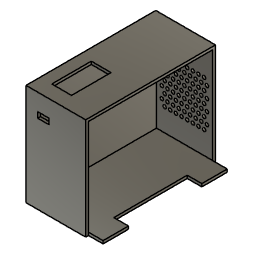
Pc v2.1 v3 (Autodesk Fusion 360 design; units mm, degrees)
Autodesk Fusion 360 part; units mm, degrees
sketch "Boceto1" plane through (0, 0, 0) normal (1, 0, 0) x (0, 1, 0)
  line L0 (0, 0) -> (230, 0)
  line L1 (230, 0) -> (230, 180)
  line L2 (230, 180) -> (0, 180)
  line L3 (0, 180) -> (0, 0)
  line L4 (5, 5) -> (225, 5)
  line L5 (225, 5) -> (225, 175)
  line L6 (225, 175) -> (5, 175)
  line L7 (5, 175) -> (5, 5)
  constraint horizontal L0
  constraint vertical L1
  constraint horizontal L2
  constraint vertical L3
  constraint coincident L0.start L3.end
  constraint horizontal L4
  constraint vertical L5
  constraint horizontal L6
  constraint vertical L7
extrude "Extruir1" add sketch "Boceto1" along normal blind 100
sketch "Boceto2" plane through (0, 230, 0) normal (0, 1, 0) x (-1, 0, 0)
  line L0 (0, 0) -> (0, 180)
  line L1 (0, 180) -> (-100, 180)
  line L2 (-100, 180) -> (-100, 0)
  line L3 (-100, 0) -> (0, 0)
  circle A0 centre (-90, 115) radius 3
  circle A1 centre (-80, 115) radius 3
  circle A2 centre (-70, 115) radius 3
  circle A3 centre (-60, 115) radius 3
  circle A4 centre (-50, 115) radius 3
  circle A5 centre (-40, 115) radius 3
  circle A6 centre (-30, 115) radius 3
  circle A7 centre (-20, 115) radius 3
  circle A8 centre (-10, 115) radius 3
  circle A9 centre (-90, 115) radius 3
  circle A10 centre (-10, 115) radius 3
  circle A11 centre (-60, 115) radius 3
  circle A12 centre (-50, 115) radius 3
  circle A13 centre (-20, 115) radius 3
  circle A14 centre (-40, 115) radius 3
  circle A15 centre (-80, 115) radius 3
  circle A16 centre (-70, 115) radius 3
  circle A17 centre (-30, 115) radius 3
  circle A18 centre (-85, 105) radius 3
  circle A19 centre (-55, 105) radius 3
  circle A20 centre (-45, 105) radius 3
  circle A21 centre (-15, 105) radius 3
  circle A22 centre (-35, 105) radius 3
  circle A23 centre (-75, 105) radius 3
  circle A24 centre (-65, 105) radius 3
  circle A25 centre (-25, 105) radius 3
  circle A26 centre (-90, 95) radius 3
  circle A27 centre (-10, 95) radius 3
  circle A28 centre (-60, 95) radius 3
  circle A29 centre (-50, 95) radius 3
  circle A30 centre (-20, 95) radius 3
  circle A31 centre (-40, 95) radius 3
  circle A32 centre (-80, 95) radius 3
  circle A33 centre (-70, 95) radius 3
  circle A34 centre (-30, 95) radius 3
  circle A35 centre (-85, 85) radius 3
  circle A36 centre (-55, 85) radius 3
  circle A37 centre (-45, 85) radius 3
  circle A38 centre (-15, 85) radius 3
  circle A39 centre (-35, 85) radius 3
  circle A40 centre (-75, 85) radius 3
  circle A41 centre (-65, 85) radius 3
  circle A42 centre (-25, 85) radius 3
  circle A43 centre (-90, 75) radius 3
  circle A44 centre (-10, 75) radius 3
  circle A45 centre (-60, 75) radius 3
  circle A46 centre (-50, 75) radius 3
  circle A47 centre (-20, 75) radius 3
  circle A48 centre (-40, 75) radius 3
  circle A49 centre (-80, 75) radius 3
  circle A50 centre (-70, 75) radius 3
  circle A51 centre (-30, 75) radius 3
  circle A52 centre (-85, 65) radius 3
  circle A53 centre (-55, 65) radius 3
  circle A54 centre (-45, 65) radius 3
  circle A55 centre (-15, 65) radius 3
  circle A56 centre (-35, 65) radius 3
  circle A57 centre (-75, 65) radius 3
  circle A58 centre (-65, 65) radius 3
  circle A59 centre (-25, 65) radius 3
  circle A60 centre (-90, 55) radius 3
  circle A61 centre (-10, 55) radius 3
  circle A62 centre (-60, 55) radius 3
  circle A63 centre (-50, 55) radius 3
  circle A64 centre (-20, 55) radius 3
  circle A65 centre (-40, 55) radius 3
  circle A66 centre (-80, 55) radius 3
  circle A67 centre (-70, 55) radius 3
  circle A68 centre (-30, 55) radius 3
  circle A69 centre (-85, 45) radius 3
  circle A70 centre (-55, 45) radius 3
  circle A71 centre (-45, 45) radius 3
  circle A72 centre (-15, 45) radius 3
  circle A73 centre (-35, 45) radius 3
  circle A74 centre (-75, 45) radius 3
  circle A75 centre (-65, 45) radius 3
  circle A76 centre (-25, 45) radius 3
  circle A77 centre (-85, 125) radius 3
  circle A78 centre (-55, 125) radius 3
  circle A79 centre (-45, 125) radius 3
  circle A80 centre (-15, 125) radius 3
  circle A81 centre (-35, 125) radius 3
  circle A82 centre (-75, 125) radius 3
  circle A83 centre (-65, 125) radius 3
  circle A84 centre (-25, 125) radius 3
extrude "Extruir2" cut sketch "Boceto2" against normal blind 20 contours A0 A9 | A1 A15 | A2 A16 | A3 A11 | A4 A12 | A5 A14 | A6 A17 | A7 A13 | A8 A10 | A18 | A19 | A20 | A21 | A22 | A23 | A24 | A25 | A26 | A27 | A28 | A29 | A30 | A31 | A32 | A33 | A34 | A35 | A36 | A37 | A38 | A39 | A40 | A41 | A42 | A43 | A44 | A45 | A46 | A47 | A48 | A49 | A50 | A51 | A52 | A53 | A54 | A55 | A56 | A57 | A58 | A59 | A60 | A61 | A62 | A63 | A64 | A65 | A66 | A67 | A68 | A69 | A70 | A71 | A72 | A73 | A74 | A75 | A76 | A77 | A78 | A79 | A80 | A81 | A82 | A83 | A84
sketch "Boceto3" plane through (0, 0, 180) normal (0, 0, 1) x (-1, 0, 0)
  line L0 (0, -230) -> (0, 0)
  line L1 (0, 0) -> (-100, 0)
  line L2 (-100, 0) -> (-100, -230)
  line L3 (-100, -230) -> (0, -230)
  line L4 (-15, -25) -> (-50, -25)
  line L5 (-50, -25) -> (-50, -95)
  line L6 (-50, -95) -> (-15, -95)
  line L7 (-15, -95) -> (-15, -25)
  constraint horizontal L4
  constraint vertical L5
  constraint horizontal L6
  constraint vertical L7
sketch "Boceto4" plane through (0, 0, 180) normal (0, 0, 1) x (-1, 0, 0)
extrude "Extruir3" cut sketch "Boceto3" against normal blind 20 contours L4 L5 L6 L7
sketch "Boceto5" plane through (0, 0, 0) normal (0, -1, 0) x (1, 0, 0)
  line L0 (0, 180) -> (0, 0)
  line L1 (0, 0) -> (100, 0)
  line L2 (100, 0) -> (100, 180)
  line L3 (100, 180) -> (0, 180)
  line L4 (15, 140) -> (35, 140)
  line L5 (35, 140) -> (35, 150)
  line L6 (35, 150) -> (15, 150)
  line L7 (15, 150) -> (15, 140)
  constraint horizontal L4
  constraint vertical L5
  constraint horizontal L6
  constraint vertical L7
extrude "Extruir4" cut sketch "Boceto5" against normal blind 20 contours L4 L5 L6 L7
sketch "Boceto6" plane through (100, 0, 0) normal (1, 0, 0) x (0, 1, 0)
  line L0 (5, 5) -> (5, 175)
  line L1 (5, 175) -> (225, 175)
  line L2 (225, 175) -> (225, 5)
  line L3 (225, 5) -> (5, 5)
  line L4 (0, 180) -> (0, 0)
  line L5 (0, 0) -> (230, 0)
  line L6 (230, 0) -> (230, 180)
  line L7 (230, 180) -> (0, 180)
sketch "Boceto7" plane through (100, 0, 0) normal (1, 0, 0) x (0, 1, 0)
  line L0 (0, 0) -> (0, 5)
  line L1 (5, 5) -> (5, 0)
  line L2 (5, 0) -> (50, 0)
  line L3 (50, 0) -> (50, 5)
  line L4 (50, 5) -> (5, 5)
  line L5 (225, 5) -> (180, 5)
  line L6 (180, 5) -> (180, 0)
  line L7 (180, 0) -> (225, 0)
  line L8 (225, 0) -> (225, 5)
  dimension "d9" = 45
  constraint coincident L0.start origin
  constraint vertical L0
  constraint vertical L1
  constraint perpendicular L1 L2
  constraint perpendicular L2 L3
  constraint perpendicular L1 L4
  constraint horizontal L5
  constraint perpendicular L5 L6
  constraint perpendicular L6 L7
  constraint perpendicular L5 L8
  measures "d9" distance of L5.start L5.end
extrude "Extruir5" add sketch "Boceto7" along normal blind 23
sketch "Boceto8" plane through (0, 0, 0) normal (-1, 0, 0) x (0, -1, 0)
  line L0 (-5, 175) -> (-5, 5)
  line L1 (-5, 5) -> (-225, 5)
  line L2 (-225, 5) -> (-225, 175)
  line L3 (-225, 175) -> (-5, 175)
  line L4 (0, 0) -> (0, 180)
  line L5 (0, 180) -> (-230, 180)
  line L6 (-230, 180) -> (-230, 0)
  line L7 (-230, 0) -> (0, 0)
  line L8 (-230, 180) -> (0, 180)
  line L9 (0, 180) -> (0, 0)
  line L10 (0, 0) -> (-230, 0)
  line L11 (-230, 0) -> (-230, 180)
  constraint horizontal L8
  constraint vertical L9
  constraint horizontal L10
  constraint vertical L11
  constraint coincident L4.start L7.end
  constraint coincident L5.end L6.start
extrude "Extruir6" add sketch "Boceto8" against normal blind 0.5 contours L0 L1 L2 L3
sketch "Boceto9" plane through (0, 0, 0) normal (-1, 0, 0) x (0, -1, 0)
  line L0 (0, 0) -> (0, 180)
  line L1 (0, 180) -> (-230, 180)
  line L2 (-230, 180) -> (-230, 0)
  line L3 (-230, 0) -> (0, 0)
  line L4 (-220, 170) -> (-215, 175)
  line L5 (-215, 175) -> (-210, 170)
  line L6 (-210, 170) -> (-215, 165)
  line L7 (-215, 165) -> (-220, 170)
  line L8 (-225, 165) -> (-220, 160)
  line L9 (-220, 160) -> (-225, 155)
  line L10 (-225, 155) -> (-225, 165)
  constraint perpendicular L5 L6
  constraint perpendicular L4 L8
  constraint perpendicular L8 L9
  constraint vertical L10
scale "Escala1" factor 1 about (100, 0, 180) bodies 1
scale "Escala2" factor 0.87 about (100, 0, 180) bodies 1
move_body "Desplazar1" bodies 1 to x (1, 0, 0) y (0, 1, 0) z (0, 0, 1) at (0, 0, -20)
extrude "Extruir7" add 1 faces at (120.01, 17.4, 6.3) along direction (1, 0, 0) blind 2.5
extrude "Extruir8" add 1 faces at (120.01, 169.65, 6.3) along direction (1, 0, 0) blind 2.5
extrude "Extruir9" add 1 faces at (13, 133.4, 107.8) along direction (-1, 0, 0) blind 3
extrude "Extruir10" add 1 faces at (10, 133.4, 107.8) along direction (-1, 0, 0) blind 2
